Autodesk Fusion 360 part; units mm, degrees
note: some values were not read from the file. Set by a fixed rule: which sketch regions a step uses.
(part 6 of 8)
  line L4057 (-109.4829, 14.0343) -> (-108.6825, 14.0343)
  line L4058 (252.529, -8.6909) -> (249.732, -8.6909)
  line L4059 (256.681, -6.1416) -> (255.761, -6.1416)
  line L4060 (-75.345, 80.0836) -> (-76.144, 80.0836)
  line L4061 (-61.057, 41.9836) -> (-61.057, 38.8844)
  line L4062 (-108.6825, 14.0343) -> (-108.6825, 10.9337)
  line L4063 (253.129, 0.4083) -> (252.529, 0.4083)
  line L4064 (-47.283, 22.9336) -> (-48.083, 22.9336)
  line L4065 (-71.095, 67.0833) -> (-71.095, 68.0838)
  line L4066 (-65.82, 57.9344) -> (-66.62, 57.9344)
  line L4067 (-91.2764, -8.8866) -> (-91.2764, -2.6165)
  line L4068 (-148.0943, 76.9844) -> (-147.295, 76.9844)
  line L4069 (-147.295, 80.0836) -> (-148.0943, 80.0836)
  line L4070 (-56.808, 42.984) -> (-56.808, 41.9836)
  line L4071 (0.056, 81.084) -> (0.056, 80.0836)
  line L4072 (-32.482, 19.8345) -> (-32.482, 22.9336)
  line L4073 (-102.3378, -9.1167) -> (-102.3378, -8.1163)
  line L4074 (-52.045, 81.084) -> (-52.045, 80.0836)
  line L4075 (-51.532, 19.8345) -> (-51.532, 22.9336)
  line L4076 (-71.095, 68.0838) -> (-71.095, 67.0833)
  line L4077 (-147.295, 71.1844) -> (-148.0943, 71.1844)
  line L4078 (-61.057, 38.8844) -> (-61.057, 41.9836)
  line L4079 (-80.6201, 62.034) -> (-66.62, 62.034)
  line L4080 (-151.5449, 108.6602) -> (-151.5449, 105.5592)
  line L4081 (-33.283, 19.8345) -> (-32.482, 19.8345)
  line L4082 (-65.82, 52.1344) -> (-66.62, 52.1344)
  line L4083 (-151.5449, 76.9844) -> (-151.5449, 80.0836)
  line L4084 (249.732, -7.8669) -> (249.732, -8.6909)
  line L4085 (257.232, 0.4083) -> (256.23, 0.4083)
  line L4086 (-56.808, 41.9836) -> (-56.808, 42.984)
  line L4087 (-147.295, 68.0838) -> (-148.0943, 68.0838)
  line L4088 (-166.345, 99.7592) -> (-167.1443, 99.7592)
  line L4089 (-71.3829, 19.8345) -> (-71.3829, 14.0343)
  line L4090 (-66.62, 52.1344) -> (-66.62, 57.9344)
  line L4091 (-61.057, 41.9836) -> (-61.858, 41.9836)
  line L4092 (-66.62, 49.0338) -> (-66.62, 48.0333)
  line L4093 (-91.2764, 0.1836) -> (-92.1019, 0.1836)
  line L4094 (-89.551, 4.3343) -> (-89.551, 3.4138)
  line L4095 (-18.994, 71.1844) -> (-18.195, 71.1844)
  line L4096 (-123.4826, 10.9337) -> (-123.4826, 9.9333)
  line L4097 (-76.144, 68.0838) -> (-75.345, 68.0838)
  line L4098 (247.929, 0.4083) -> (247.929, -1.1159)
  line L4099 (-23.758, 42.984) -> (-37.758, 42.984)
  line L4100 (-13.945, 71.1844) -> (-13.945, 76.9844)
  line L4101 (255.761, -1.1159) -> (255.761, -2.8412)
  line L4102 (-127.7325, 14.0343) -> (-127.7325, 10.9337)
  line L4103 (249.732, -8.6909) -> (249.732, -7.8669)
  line L4104 (-147.295, 76.9844) -> (-148.0943, 76.9844)
  line L4105 (-52.333, 22.9336) -> (-52.333, 23.934)
  line L4106 (-48.083, 22.9336) -> (-48.083, 19.8345)
  line L4107 (-148.0943, 71.1844) -> (-147.295, 71.1844)
  arc A65 (-161.6635, 120.9832) -> (-163.6635, 118.9832) centre (-161.6635, 118.9832) ccw
  line L4108 (-102.3378, 4.8841) -> (-102.3378, 3.8837)
  line L4109 (-65.82, 57.9344) -> (-65.82, 61.0336)
  line L4110 (-75.345, 80.0836) -> (-75.345, 76.9844)
  line L4111 (-56.808, 33.0844) -> (-56.808, 38.8844)
  line L4112 (-171.0689, 114.1832) -> (-165.6635, 114.1832)
  line L4113 (-80.6201, 61.0336) -> (-80.6201, 62.034)
  line L4114 (-128.5329, 10.9337) -> (-127.7325, 10.9337)
  line L4115 (-66.62, 48.0333) -> (-66.62, 49.0338)
  line L4116 (-166.345, 108.6602) -> (-167.1443, 108.6602)
  line L4117 (-151.5449, 80.0836) -> (-151.5449, 76.9844)
  line L4118 (-167.1443, 105.5592) -> (-167.1443, 108.6602)
  line L4119 (-61.858, 33.0844) -> (-61.057, 33.0844)
  line L4120 (-18.195, 71.1844) -> (-18.994, 71.1844)
  line L4121 (-75.345, 68.0838) -> (-76.144, 68.0838)
  line L4122 (-152.3441, 67.0833) -> (-166.345, 67.0833)
  line L4123 (-109.4829, 9.9333) -> (-109.4829, 10.9337)
  line L4124 (-89.551, -8.8866) -> (-91.2764, -8.8866)
  line L4125 (-71.095, 71.1844) -> (-71.8941, 71.1844)
  line L4126 (-66.62, 61.0336) -> (-65.82, 61.0336)
  line L4127 (-66.62, 62.034) -> (-66.62, 61.0336)
  line L4128 (-123.4826, 9.9333) -> (-109.4829, 9.9333)
  line L4129 (-66.62, 57.9344) -> (-65.82, 57.9344)
  line L4130 (-71.095, 80.0836) -> (-71.8941, 80.0836)
  line L4131 (-167.1443, 99.7592) -> (-166.345, 99.7592)
  line L4132 (-18.195, 68.0838) -> (-18.994, 68.0838)
  line L4133 (-101.5387, 0.7845) -> (-101.5387, 3.8837)
  line L4134 (-102.3378, 0.7845) -> (-101.5387, 0.7845)
  line L4135 (252.529, 0.4083) -> (253.129, 0.4083)
  line L4136 (-18.994, 71.1844) -> (-18.994, 76.9844)
  line L4137 (-124.283, 14.0343) -> (-123.4826, 14.0343)
  line L4138 (-37.758, 28.9833) -> (-23.758, 28.9833)
  line L4139 (256.23, -0.391) -> (253.129, -0.391)
  line L4140 (-61.858, 41.9836) -> (-61.858, 42.984)
  line L4141 (-166.345, 95.6582) -> (-166.345, 96.6592)
  line L4142 (-61.858, 38.8844) -> (-61.057, 38.8844)
  line L4143 (-166.345, 109.6602) -> (-166.345, 108.6602)
  line L4144 (-23.758, 28.9833) -> (-37.758, 28.9833)
  line L4145 (-14.744, 68.0838) -> (-13.945, 68.0838)
  line L4146 (-56.808, 41.9836) -> (-57.608, 41.9836)
  line L4147 (-167.1443, 99.7592) -> (-167.1443, 96.6592)
  line L4148 (-91.2764, -2.6165) -> (-92.1019, -2.6165)
  line L4149 (-66.333, 19.8345) -> (-66.333, 14.0343)
  line L4150 (-75.345, 71.1844) -> (-75.345, 68.0838)
  line L4151 (-37.758, 42.984) -> (-23.758, 42.984)
  line L4152 (-18.994, 68.0838) -> (-18.195, 68.0838)
  line L4153 (-108.6825, 10.9337) -> (-108.6825, 14.0343)
  line L4154 (-123.4826, 14.0343) -> (-124.283, 14.0343)
  line L4155 (-66.62, 52.1344) -> (-65.82, 52.1344)
  line L4156 (-56.808, 38.8844) -> (-56.808, 33.0844)
  line L4157 (-76.144, 68.0838) -> (-76.144, 67.0833)
  line L4158 (-163.6635, 118.9832) -> (-163.6635, 116.1832)
  line L4159 (-166.345, 108.6602) -> (-166.345, 109.6602)
  line L4160 (-57.608, 33.0844) -> (-56.808, 33.0844)
  arc A66 (-165.6635, 114.1832) -> (-163.6635, 116.1832) centre (-165.6635, 116.1832) ccw
  line L4161 (-152.3441, 68.0838) -> (-151.5449, 68.0838)
  line L4162 (-52.333, 19.8345) -> (-52.333, 14.0343)
  line L4163 (-66.62, 49.0338) -> (-65.82, 49.0338)
  line L4164 (-18.195, 76.9844) -> (-18.195, 80.0836)
  line L4165 (-18.195, 80.0836) -> (-18.195, 76.9844)
  line L4166 (-127.7325, 10.9337) -> (-127.7325, 14.0343)
  line L4167 (-71.3829, 14.0343) -> (-71.3829, 19.8345)
  line L4168 (-56.808, 38.8844) -> (-57.608, 38.8844)
  line L4169 (-71.8941, 76.9844) -> (-71.8941, 80.0836)
  line L4170 (-166.345, 96.6592) -> (-166.345, 95.6582)
  line L4171 (-102.3378, 3.8837) -> (-102.3378, 4.8841)
  line L4172 (-102.3378, -5.0157) -> (-101.5387, -5.0157)
  line L4173 (-124.283, 10.9337) -> (-123.4826, 10.9337)
  line L4174 (-75.345, 71.1844) -> (-76.144, 71.1844)
  line L4175 (-123.4826, 10.9337) -> (-124.283, 10.9337)
  line L4176 (-71.8941, 68.0838) -> (-71.095, 68.0838)
  line L4177 (-66.62, 61.0336) -> (-66.62, 62.034)
  line L4178 (-102.3378, -5.0157) -> (-102.3378, 0.7845)
  line L4179 (-9.469, 105.5592) -> (-8.67, 105.5592)
  line L4180 (-90.4329, 14.0343) -> (-90.4329, 19.8345)
  line L4181 (-9.469, 52.1344) -> (-9.469, 57.9344)
  line L4182 (5.105, 68.0838) -> (4.306, 68.0838)
  line L4183 (-42.007, 38.8844) -> (-42.808, 38.8844)
  line L4184 (243.459, -2.8412) -> (242.482, -2.8412)
  line L4185 (-9.469, 108.6602) -> (-9.469, 109.6602)
  line L4186 (-104.4326, 9.9333) -> (-90.4329, 9.9333)
  line L4187 (-146.7824, 49.0338) -> (-146.7824, 52.1344)
  line L4188 (256.23, 14.4091) -> (257.232, 14.4091)
  line L4189 (-128.2451, 108.6602) -> (-129.0441, 108.6602)
  line L4190 (-90.4329, 14.0343) -> (-89.6325, 14.0343)
  line L4191 (-8.67, 105.5592) -> (-9.469, 105.5592)
  line L4192 (-128.2451, 96.6592) -> (-128.2451, 95.6582)
  line L4193 (-147.583, 57.9344) -> (-146.7824, 57.9344)
  line L4194 (253.129, 15.2084) -> (256.23, 15.2084)
  line L4195 (256.23, 15.2084) -> (253.129, 15.2084)
  line L4196 (-52.333, 9.9333) -> (-66.333, 9.9333)
  line L4197 (244.232, 0.4083) -> (244.232, -0.391)
  line L4198 (-128.2451, 95.6582) -> (-128.2451, 96.6592)
  line L4199 (0.855, 71.1844) -> (0.855, 68.0838)
  line L4200 (0.056, 81.084) -> (-13.945, 81.084)
  line L4201 (242.482, -6.1416) -> (242.482, -2.8412)
  line L4202 (-147.583, 52.1344) -> (-147.583, 57.9344)
  line L4203 (-71.095, 67.0833) -> (-57.094, 67.0833)
  line L4204 (-9.469, 52.1344) -> (-8.67, 52.1344)
  line L4205 (-146.7824, 52.1344) -> (-146.7824, 49.0338)
  line L4206 (252.529, 15.9333) -> (255.761, 15.9333)
  line L4207 (-42.808, 42.984) -> (-42.808, 41.9836)
  line L4208 (-42.808, 28.9833) -> (-42.808, 29.9838)
  line L4209 (244.232, -0.391) -> (247.333, -0.391)
  line L4210 (-128.2451, 99.7592) -> (-129.0441, 99.7592)
  line L4211 (-44.901, -4.4162) -> (-84.5267, -4.4162)
  line L4212 (-90.4329, 10.9337) -> (-90.4329, 9.9333)
  line L4213 (5.105, 71.1844) -> (4.306, 71.1844)
  line L4214 (-9.469, 61.0336) -> (-8.67, 61.0336)
  line L4215 (-116.3388, 4.8841) -> (-102.3378, 4.8841)
  line L4216 (-42.007, 29.9838) -> (-42.808, 29.9838)
  line L4217 (-128.2451, 96.6592) -> (-129.0441, 96.6592)
  line L4218 (238.979, -5.0157) -> (238.182, -5.0157)
  line L4219 (5.105, 68.0838) -> (5.105, 67.0833)
  line L4220 (-90.4329, 9.9333) -> (-104.4326, 9.9333)
  line L4221 (-57.094, 81.084) -> (-71.095, 81.084)
  line L4222 (-8.67, 61.0336) -> (-9.469, 61.0336)
  line L4223 (243.459, -1.1159) -> (247.929, -1.1159)
  line L4224 (255.761, 15.9333) -> (252.529, 15.9333)
  line L4225 (-42.808, 33.0844) -> (-42.007, 33.0844)
  line L4226 (-90.4329, 10.9337) -> (-89.6325, 10.9337)
  line L4227 (-147.583, 52.1344) -> (-146.7824, 52.1344)
  line L4228 (-105.233, 10.9337) -> (-105.233, 14.0343)
  line L4229 (-129.0441, 108.6602) -> (-128.2451, 108.6602)
  line L4230 (-129.0441, 99.7592) -> (-128.2451, 99.7592)
  line L4231 (-133.294, 67.0833) -> (-147.295, 67.0833)
  line L4232 (-147.583, 62.034) -> (-147.583, 61.0336)
  line L4233 (-146.7824, 61.0336) -> (-147.583, 61.0336)
  line L4234 (5.105, 80.0836) -> (4.306, 80.0836)
  line L4235 (-57.094, 67.0833) -> (-71.095, 67.0833)
  line L4236 (-8.67, 57.9344) -> (-9.469, 57.9344)
  line L4237 (243.459, -6.1416) -> (242.482, -6.1416)
  line L4238 (-42.808, 29.9838) -> (-42.808, 28.9833)
  line L4239 (252.529, 14.4091) -> (253.129, 14.4091)
  line L4240 (5.105, 80.0836) -> (5.105, 81.084)
  line L4241 (-116.3388, -9.1167) -> (-102.3378, -9.1167)
  line L4242 (-42.007, 41.9836) -> (-42.808, 41.9836)
  line L4243 (-146.7824, 57.9344) -> (-146.7824, 61.0336)
  line L4244 (242.482, -2.8412) -> (243.459, -2.8412)
  line L4245 (-129.0441, 96.6592) -> (-128.2451, 96.6592)
  line L4246 (244.232, -0.391) -> (244.232, 0.4083)
  line L4247 (-102.3378, -9.1167) -> (-116.3388, -9.1167)
  line L4248 (243.459, -1.1159) -> (243.459, -2.8412)
  line L4249 (-104.4326, 10.9337) -> (-105.233, 10.9337)
  line L4250 (238.182, -5.0157) -> (238.182, 0.7845)
  line L4251 (-146.7824, 52.1344) -> (-147.583, 52.1344)
  line L4252 (-42.808, 38.8844) -> (-42.808, 33.0844)
  line L4253 (238.979, -8.1163) -> (238.182, -8.1163)
  line L4254 (-129.0441, 99.7592) -> (-129.0441, 96.6592)
  line L4255 (-128.2451, 105.5592) -> (-129.0441, 105.5592)
  line L4256 (-89.6325, 10.9337) -> (-89.6325, 14.0343)
  line L4257 (-90.4329, 9.9333) -> (-90.4329, 10.9337)
  line L4258 (242.482, -2.8412) -> (242.482, -6.1416)
  line L4259 (-128.2451, 99.7592) -> (-128.2451, 105.5592)
  line L4260 (-128.2451, 108.6602) -> (-128.2451, 109.6602)
  line L4261 (-146.7824, 61.0336) -> (-146.7824, 57.9344)
  line L4262 (5.105, 81.084) -> (5.105, 80.0836)
  line L4263 (-42.007, 33.0844) -> (-42.808, 33.0844)
  line L4264 (238.182, -8.1163) -> (238.182, -9.1167)
  line L4265 (-42.808, 33.0844) -> (-42.808, 38.8844)
  line L4266 (0.855, 76.9844) -> (0.855, 80.0836)
  line L4267 (-147.295, 67.0833) -> (-133.294, 67.0833)
  line L4268 (-71.095, 81.084) -> (-57.094, 81.084)
  line L4269 (-147.583, 48.0333) -> (-147.583, 49.0338)
  line L4270 (-9.469, 57.9344) -> (-8.67, 57.9344)
  line L4271 (-57.094, 68.0838) -> (-57.094, 67.0833)
  line L4272 (-52.844, 76.9844) -> (-52.045, 76.9844)
  line L4273 (-147.583, 61.0336) -> (-146.7824, 61.0336)
  line L4274 (-166.345, 109.6602) -> (-152.3441, 109.6602)
  line L4275 (-129.0441, 96.6592) -> (-129.0441, 99.7592)
  line L4276 (-104.4326, 14.0343) -> (-105.233, 14.0343)
  line L4277 (-147.295, 81.084) -> (-133.294, 81.084)
  line L4278 (-129.0441, 105.5592) -> (-129.0441, 108.6602)
  line L4279 (0.056, 76.9844) -> (0.855, 76.9844)
  line L4280 (-52.844, 80.0836) -> (-52.045, 80.0836)
  line L4281 (253.129, -0.391) -> (253.129, 0.4083)
  line L4282 (-128.2451, 105.5592) -> (-128.2451, 99.7592)
  line L4283 (-84.5267, -4.4162) -> (-44.901, -4.4162)
  line L4284 (-162.3832, 57.9344) -> (-162.3832, 61.0336)
  line L4285 (-57.094, 76.9844) -> (-57.094, 71.1844)
  line L4286 (-57.094, 67.0833) -> (-57.094, 68.0838)
  line L4287 (-133.294, 81.084) -> (-147.295, 81.084)
  line L4288 (-162.3832, 52.1344) -> (-162.3832, 49.0338)
  line L4289 (-162.3832, 61.0336) -> (-162.3832, 57.9344)
  line L4290 (-128.2451, 109.6602) -> (-128.2451, 108.6602)
  line L4291 (-129.0441, 108.6602) -> (-129.0441, 105.5592)
  line L4292 (244.232, 0.4083) -> (243.23, 0.4083)
  line L4293 (-89.6325, 14.0343) -> (-89.6325, 10.9337)
  line L4294 (-52.844, 76.9844) -> (-52.844, 80.0836)
  line L4295 (247.333, -0.391) -> (244.232, -0.391)
  line L4296 (-89.6325, 14.0343) -> (-90.4329, 14.0343)
  line L4297 (-152.3441, 109.6602) -> (-152.3441, 108.6602)
  line L4298 (-162.3832, 49.0338) -> (-162.3832, 52.1344)
  line L4299 (-8.67, 57.9344) -> (-8.67, 61.0336)
  line L4300 (-105.233, 14.0343) -> (-104.4326, 14.0343)
  line L4301 (-151.5449, 96.6592) -> (-151.5449, 99.7592)
  line L4302 (238.182, 4.8841) -> (238.182, 3.8837)
  line L4303 (238.182, 0.7845) -> (238.182, -5.0157)
  line L4304 (-152.3441, 105.5592) -> (-151.5449, 105.5592)
  line L4305 (-152.3441, 96.6592) -> (-152.3441, 95.6582)
  line L4306 (-52.844, 71.1844) -> (-52.844, 68.0838)
  line L4307 (242.482, -6.1416) -> (243.459, -6.1416)
  line L4308 (4.306, 71.1844) -> (5.105, 71.1844)
  line L4309 (-162.3832, 52.1344) -> (-161.5825, 52.1344)
  line L4310 (0.056, 67.0833) -> (0.056, 68.0838)
  line L4311 (243.459, -6.1416) -> (243.459, -7.8669)
  line L4312 (0.056, 71.1844) -> (0.855, 71.1844)
  line L4313 (-9.469, 62.034) -> (-9.469, 61.0336)
  line L4314 (243.459, -2.8412) -> (243.459, -1.1159)
  line L4315 (-152.3441, 80.0836) -> (-152.3441, 81.084)
  line L4316 (238.979, 0.7845) -> (238.182, 0.7845)
  line L4317 (4.306, 68.0838) -> (5.105, 68.0838)
  line L4318 (-161.5825, 61.0336) -> (-162.3832, 61.0336)
  line L4319 (238.182, 3.8837) -> (238.979, 3.8837)
  line L4320 (-152.3441, 105.5592) -> (-152.3441, 99.7592)
  line L4321 (-57.094, 76.9844) -> (-56.295, 76.9844)
  line L4322 (-162.3832, 49.0338) -> (-161.5825, 49.0338)
  line L4323 (-52.844, 71.1844) -> (-52.045, 71.1844)
  line L4324 (-52.045, 80.0836) -> (-52.844, 80.0836)
  line L4325 (-151.5449, 108.6602) -> (-152.3441, 108.6602)
  line L4326 (255.761, -6.1416) -> (256.681, -6.1416)
  line L4327 (-151.5449, 105.5592) -> (-151.5449, 108.6602)
  line L4328 (256.681, -2.8412) -> (255.761, -2.8412)
  line L4329 (-9.469, 61.0336) -> (-9.469, 62.034)
  line L4330 (-161.5825, 49.0338) -> (-162.3832, 49.0338)
  line L4331 (-162.3832, 57.9344) -> (-161.5825, 57.9344)
  line L4332 (-57.094, 81.084) -> (-57.094, 80.0836)
  line L4333 (243.23, 0.4083) -> (244.232, 0.4083)
  line L4334 (-9.469, 57.9344) -> (-9.469, 52.1344)
  line L4335 (-56.295, 68.0838) -> (-56.295, 71.1844)
  line L4336 (-161.5825, 61.0336) -> (-161.5825, 62.034)
  line L4337 (238.979, -5.0157) -> (238.979, -8.1163)
  line L4338 (238.979, -8.1163) -> (238.979, -5.0157)
  line L4339 (-152.3441, 95.6582) -> (-152.3441, 96.6592)
  line L4340 (252.529, -8.6909) -> (252.529, -7.8669)
  line L4341 (4.306, 80.0836) -> (4.306, 76.9844)
  line L4342 (-152.3441, 96.6592) -> (-151.5449, 96.6592)
  line L4343 (-161.5825, 52.1344) -> (-162.3832, 52.1344)
  line L4344 (243.459, -7.8669) -> (243.459, -6.1416)
  line L4345 (-151.5449, 96.6592) -> (-152.3441, 96.6592)
  line L4346 (-161.5825, 57.9344) -> (-161.5825, 52.1344)
  line L4347 (-56.295, 71.1844) -> (-57.094, 71.1844)
  line L4348 (255.761, -7.8669) -> (255.761, -6.1416)
  line L4349 (238.979, 3.8837) -> (238.182, 3.8837)
  line L4350 (-151.5449, 71.1844) -> (-152.3441, 71.1844)
  line L4351 (-161.5825, 62.034) -> (-147.583, 62.034)
  line L4352 (-52.045, 76.9844) -> (-52.045, 71.1844)
  line L4353 (-52.333, 23.934) -> (-52.333, 22.9336)
  line L4354 (-147.583, 48.0333) -> (-161.5825, 48.0333)
  line L4355 (-166.345, 95.6582) -> (-152.3441, 95.6582)
  line L4356 (-52.045, 71.1844) -> (-52.844, 71.1844)
  line L4357 (238.182, -5.0157) -> (238.979, -5.0157)
  line L4358 (4.306, 76.9844) -> (5.105, 76.9844)
  line L4359 (-161.5825, 48.0333) -> (-147.583, 48.0333)
  line L4360 (238.979, 3.8837) -> (238.979, 0.7845)
  line L4361 (-152.3441, 95.6582) -> (-166.345, 95.6582)
  line L4362 (252.529, -7.8669) -> (255.761, -7.8669)
  line L4363 (-145.2635, 118.9832) -> (-145.2635, 116.1832)
  line L4364 (247.929, 0.4083) -> (247.333, 0.4083)
  line L4365 (256.23, 0.4083) -> (256.23, -0.391)
  line L4366 (-51.532, 19.8345) -> (-52.333, 19.8345)
  line L4367 (0.855, 68.0838) -> (0.855, 71.1844)
  line L4368 (-147.583, 62.034) -> (-161.5825, 62.034)
  line L4369 (-151.5449, 105.5592) -> (-152.3441, 105.5592)
  line L4370 (-47.283, 23.934) -> (-47.283, 22.9336)
  line L4371 (247.333, 0.4083) -> (247.929, 0.4083)
  line L4372 (-161.5825, 49.0338) -> (-161.5825, 48.0333)
  line L4373 (4.306, 80.0836) -> (5.105, 80.0836)
  line L4374 (-57.094, 80.0836) -> (-57.094, 81.084)
  line L4375 (-51.532, 22.9336) -> (-51.532, 19.8345)
  line L4376 (-161.5825, 57.9344) -> (-162.3832, 57.9344)
  line L4377 (4.306, 68.0838) -> (4.306, 71.1844)
  line L4378 (-152.3441, 80.0836) -> (-151.5449, 80.0836)
  line L4379 (-32.482, 22.9336) -> (-32.482, 19.8345)
  line L4380 (-52.844, 80.0836) -> (-52.844, 76.9844)
  line L4381 (-66.333, 9.9333) -> (-52.333, 9.9333)
  line L4382 (-161.5825, 48.0333) -> (-161.5825, 49.0338)
  line L4383 (-156.5635, 120.9832) -> (-157.3635, 120.9832)
  line L4384 (0.056, 71.1844) -> (0.056, 76.9844)
  line L4385 (-52.045, 68.0838) -> (-52.844, 68.0838)
  arc A67 (-145.2635, 116.1832) -> (-143.2635, 114.1832) centre (-143.2635, 116.1832) ccw
  line L4386 (-162.3832, 61.0336) -> (-161.5825, 61.0336)
  line L4387 (-148.0943, 68.0838) -> (-147.295, 68.0838)
  line L4388 (-147.2635, 120.9832) -> (-161.6635, 120.9832)
  line L4389 (5.105, 67.0833) -> (5.105, 68.0838)
  line L4390 (252.529, -1.1159) -> (252.529, 0.4083)
  line L4391 (256.681, -6.1416) -> (256.681, -2.8412)
  line L4392 (253.129, -0.391) -> (256.23, -0.391)
  line L4393 (-56.295, 68.0838) -> (-57.094, 68.0838)
  line L4394 (5.105, 76.9844) -> (5.105, 71.1844)
  line L4395 (255.761, -2.8412) -> (255.761, -1.1159)
  line L4396 (-47.283, 19.8345) -> (-48.083, 19.8345)
  line L4397 (-80.6201, 57.9344) -> (-81.4205, 57.9344)
  line L4398 (0.855, 68.0838) -> (0.056, 68.0838)
  line L4399 (256.23, 0.4083) -> (257.232, 0.4083)
  line L4400 (-161.5825, 52.1344) -> (-161.5825, 57.9344)
  line L4401 (-52.844, 68.0838) -> (-52.045, 68.0838)
  line L4402 (-33.283, 22.9336) -> (-32.482, 22.9336)
  line L4403 (-101.5387, 3.8837) -> (-101.5387, 0.7845)
  line L4404 (-152.3441, 109.6602) -> (-166.345, 109.6602)
  line L4405 (-152.3441, 108.6602) -> (-152.3441, 109.6602)
  line L4406 (0.855, 80.0836) -> (0.855, 76.9844)
  line L4407 (-147.295, 67.0833) -> (-147.295, 68.0838)
  line L4408 (-52.333, 19.8345) -> (-51.532, 19.8345)
  line L4409 (-52.045, 80.0836) -> (-52.045, 81.084)
  line L4410 (-52.045, 76.9844) -> (-52.844, 76.9844)
  line L4411 (-89.551, -9.8664) -> (-89.551, -8.8866)
  line L4412 (-52.333, 22.9336) -> (-51.532, 22.9336)
  line L4413 (-56.295, 80.0836) -> (-57.094, 80.0836)
  line L4414 (252.529, 0.4083) -> (252.529, -1.1159)
  line L4415 (256.681, -2.8412) -> (256.681, -6.1416)
  line L4416 (5.105, 76.9844) -> (4.306, 76.9844)
  line L4417 (5.105, 71.1844) -> (5.105, 76.9844)
  line L4418 (-147.295, 81.084) -> (-147.295, 80.0836)
  line L4419 (-56.295, 76.9844) -> (-56.295, 80.0836)
  line L4420 (247.333, 0.4083) -> (247.333, -0.391)
  line L4421 (-92.1019, -2.6165) -> (-91.2764, -2.6165)
  line L4422 (-89.551, -8.8866) -> (-89.551, -9.8664)
  line L4423 (-151.5449, 99.7592) -> (-152.3441, 99.7592)
  line L4424 (-161.5825, 62.034) -> (-161.5825, 61.0336)
  line L4425 (-151.5449, 71.1844) -> (-151.5449, 68.0838)
  circle A68 centre (-156.9635, 117.5832) radius 1.7
  line L4426 (-13.945, 67.0833) -> (0.056, 67.0833)
  line L4427 (252.529, -1.1159) -> (255.761, -1.1159)
  line L4428 (-102.3378, 4.8841) -> (-116.3388, 4.8841)
  line L4429 (-33.283, 22.9336) -> (-33.283, 23.934)
  line L4430 (0.056, 76.9844) -> (0.056, 71.1844)
  line L4431 (-48.083, 22.9336) -> (-47.283, 22.9336)
  line L4432 (-147.295, 76.9844) -> (-147.295, 71.1844)
  circle A69 centre (-156.9635, 117.5832) radius 1.7
  line L4433 (-47.283, 14.0343) -> (-48.083, 14.0343)
  line L4434 (-32.482, 14.0343) -> (-32.482, 10.9337)
  line L4435 (-52.333, 9.9333) -> (-52.333, 10.9337)
  line L4436 (-45.702, -8.1163) -> (-44.901, -8.1163)
  line L4437 (-44.901, 3.8837) -> (-44.901, 4.8841)
  line L4438 (-44.901, -8.1163) -> (-44.901, -9.1167)
  line L4439 (-48.083, 14.0343) -> (-47.283, 14.0343)
  line L4440 (-45.702, 0.7845) -> (-44.901, 0.7845)
  line L4441 (-32.482, 10.9337) -> (-33.283, 10.9337)
  line L4442 (-45.702, -8.1163) -> (-45.702, -5.0157)
  line L4443 (-32.482, 14.0343) -> (-33.283, 14.0343)
  line L4444 (-48.083, 14.0343) -> (-48.083, 10.9337)
  line L4445 (-44.901, 3.8837) -> (-45.702, 3.8837)
  line L4446 (-44.901, -4.4162) -> (-44.901, -5.0157)
  line L4447 (-45.702, -5.0157) -> (-45.702, -8.1163)
  line L4448 (-44.901, 4.8841) -> (-44.901, 3.8837)
  line L4449 (-48.083, 10.9337) -> (-48.083, 14.0343)
  line L4450 (-44.901, 0.1836) -> (-44.901, 0.7845)
  line L4451 (-44.901, 0.7845) -> (-44.901, 0.1836)
  line L4452 (-45.702, 0.7845) -> (-45.702, 3.8837)
  line L4453 (-61.858, 38.8844) -> (-61.858, 33.0844)
  line L4454 (-61.858, 42.984) -> (-61.858, 41.9836)
  line L4455 (-102.3378, -8.1163) -> (-101.5387, -8.1163)
  line L4456 (-101.5387, 0.7845) -> (-102.3378, 0.7845)
  line L4457 (-166.345, 99.7592) -> (-166.345, 105.5592)
  line L4458 (-13.945, 68.0838) -> (-14.744, 68.0838)
  line L4459 (-61.858, 41.9836) -> (-61.057, 41.9836)
  line L4460 (-166.345, 76.9844) -> (-166.345, 71.1844)
  line L4461 (-76.144, 71.1844) -> (-75.345, 71.1844)
  line L4462 (-61.057, 33.0844) -> (-61.858, 33.0844)
  line L4463 (-166.345, 80.0836) -> (-166.345, 81.084)
  line L4464 (-123.4826, 9.9333) -> (-123.4826, 10.9337)
  line L4465 (-166.345, 81.084) -> (-166.345, 80.0836)
  line L4466 (-109.4829, 9.9333) -> (-123.4826, 9.9333)
  line L4467 (-13.945, 76.9844) -> (-13.945, 71.1844)
  line L4468 (-76.144, 80.0836) -> (-76.144, 81.084)
  line L4469 (-14.744, 68.0838) -> (-14.744, 71.1844)
  line L4470 (-66.333, 14.0343) -> (-66.333, 19.8345)
  line L4471 (-126.1517, -5.0157) -> (-126.1517, 0.7845)
  line L4472 (-166.345, 105.5592) -> (-166.345, 99.7592)
  line L4473 (-167.1443, 96.6592) -> (-166.345, 96.6592)
  line L4474 (-125.3512, 3.8837) -> (-125.3512, 0.7845)
  line L4475 (-125.3512, 3.8837) -> (-126.1517, 3.8837)
  line L4476 (-166.345, 67.0833) -> (-152.3441, 67.0833)
  line L4477 (-57.608, 41.9836) -> (-57.608, 38.8844)
  line L4478 (-91.2764, 3.4138) -> (-91.2764, 0.1836)
  line L4479 (-13.945, 68.0838) -> (-13.945, 67.0833)
  line L4480 (-92.1019, 0.1836) -> (-92.1019, -2.6165)
  line L4481 (-80.6201, 62.034) -> (-80.6201, 61.0336)
  line L4482 (-167.1443, 105.5592) -> (-166.345, 105.5592)
  line L4483 (-151.5449, 76.9844) -> (-152.3441, 76.9844)
  line L4484 (-127.7325, 14.0343) -> (-128.5329, 14.0343)
  line L4485 (-101.5387, 3.8837) -> (-102.3378, 3.8837)
  line L4486 (-76.144, 71.1844) -> (-76.144, 76.9844)
  line L4487 (-13.945, 81.084) -> (0.056, 81.084)
  line L4488 (-80.6201, 48.0333) -> (-66.62, 48.0333)
  line L4489 (-13.945, 80.0836) -> (-14.744, 80.0836)
  line L4490 (-128.5329, 10.9337) -> (-128.5329, 9.9333)
  line L4491 (-124.283, 14.0343) -> (-124.283, 10.9337)
  line L4492 (-75.345, 76.9844) -> (-76.144, 76.9844)
  line L4493 (-61.057, 38.8844) -> (-61.858, 38.8844)
  line L4494 (-166.345, 96.6592) -> (-167.1443, 96.6592)
  line L4495 (-166.345, 76.9844) -> (-167.1443, 76.9844)
  line L4496 (-167.1443, 108.6602) -> (-167.1443, 105.5592)
  line L4497 (-109.4829, 10.9337) -> (-108.6825, 10.9337)
  line L4498 (-128.5329, 14.0343) -> (-127.7325, 14.0343)
  line L4499 (-167.1443, 108.6602) -> (-166.345, 108.6602)
  line L4500 (-101.5387, -5.0157) -> (-102.3378, -5.0157)
  line L4501 (-56.808, 33.0844) -> (-57.608, 33.0844)
  line L4502 (-126.1517, -5.0157) -> (-125.3512, -5.0157)
  line L4503 (-109.4829, 10.9337) -> (-109.4829, 9.9333)
  line L4504 (-76.144, 80.0836) -> (-75.345, 80.0836)
  line L4505 (-76.144, 81.084) -> (-76.144, 80.0836)
  line L4506 (-91.2764, -8.8866) -> (-89.551, -8.8866)
  line L4507 (-117.1378, -8.1163) -> (-116.3388, -8.1163)
  line L4508 (-117.1378, 0.7845) -> (-116.3388, 0.7845)
  line L4509 (-167.1443, 96.6592) -> (-167.1443, 99.7592)
  line L4510 (-57.608, 38.8844) -> (-56.808, 38.8844)
  line L4511 (-71.095, 76.9844) -> (-71.8941, 76.9844)
  line L4512 (-18.994, 76.9844) -> (-18.195, 76.9844)
  line L4513 (-102.3378, -8.1163) -> (-102.3378, -9.1167)
  line L4514 (-13.945, 81.084) -> (-13.945, 80.0836)
  line L4515 (-89.551, 3.4138) -> (-89.551, 4.3343)
  line L4516 (-167.1443, 80.0836) -> (-167.1443, 76.9844)
  line L4517 (-14.744, 80.0836) -> (-13.945, 80.0836)
  line L4518 (-167.1443, 76.9844) -> (-167.1443, 80.0836)
  line L4519 (-57.608, 38.8844) -> (-57.608, 41.9836)
  line L4520 (-128.5329, 9.9333) -> (-128.5329, 10.9337)
  line L4521 (-47.283, 19.8345) -> (-47.283, 14.0343)
  line L4522 (0.056, 80.0836) -> (0.855, 80.0836)
  line L4523 (-18.994, 80.0836) -> (-18.195, 80.0836)
  line L4524 (-125.3512, -8.1163) -> (-126.1517, -8.1163)
  line L4525 (-125.3512, 0.7845) -> (-126.1517, 0.7845)
  line L4526 (-57.608, 41.9836) -> (-56.808, 41.9836)
  line L4527 (-85.3826, 14.0343) -> (-85.3826, 19.8345)
  line L4528 (-101.5387, -8.1163) -> (-101.5387, -5.0157)
  line L4529 (-127.7325, 10.9337) -> (-128.5329, 10.9337)
  line L4530 (-85.6704, 49.0338) -> (-84.87, 49.0338)
  line L4531 (-71.095, 80.0836) -> (-71.095, 81.084)
  line L4532 (-71.8941, 71.1844) -> (-71.095, 71.1844)
  line L4533 (-71.8941, 68.0838) -> (-71.8941, 71.1844)
  line L4534 (-75.345, 76.9844) -> (-75.345, 80.0836)
  line L4535 (-61.858, 33.0844) -> (-61.858, 38.8844)
  line L4536 (-33.283, 14.0343) -> (-33.283, 19.8345)
  line L4537 (-71.8941, 76.9844) -> (-71.095, 76.9844)
  line L4538 (-166.345, 105.5592) -> (-167.1443, 105.5592)
  line L4539 (-18.195, 71.1844) -> (-18.195, 68.0838)
  line L4540 (-166.345, 81.084) -> (-152.3441, 81.084)
  line L4541 (-166.345, 68.0838) -> (-167.1443, 68.0838)
  line L4542 (-167.1443, 76.9844) -> (-166.345, 76.9844)
  line L4543 (-163.3635, 114.1832) -> (-165.0689, 114.1832)
  line L4544 (-85.6704, 48.0333) -> (-85.6704, 49.0338)
  line L4545 (-124.283, 10.9337) -> (-124.283, 14.0343)
  line L4546 (-18.994, 67.0833) -> (-18.994, 68.0838)
  line L4547 (-28.233, 14.0343) -> (-28.233, 19.8345)
  line L4548 (-84.87, 61.0336) -> (-85.6704, 61.0336)
  line L4549 (-71.095, 68.0838) -> (-71.8941, 68.0838)
  line L4550 (-71.095, 71.1844) -> (-71.095, 76.9844)
  line L4551 (-76.144, 67.0833) -> (-76.144, 68.0838)
  line L4552 (-29.033, 14.0343) -> (-28.233, 14.0343)
  line L4553 (-167.1443, 71.1844) -> (-167.1443, 68.0838)
  line L4554 (-84.87, 52.1344) -> (-85.6704, 52.1344)
  line L4555 (-117.1378, -5.0157) -> (-117.1378, -8.1163)
  line L4556 (-166.345, 67.0833) -> (-166.345, 68.0838)
  line L4557 (-126.1517, 3.8837) -> (-126.1517, 4.8841)
  line L4558 (-47.283, 14.0343) -> (-47.283, 19.8345)
  line L4559 (-80.6201, 57.9344) -> (-80.6201, 52.1344)
  line L4560 (-116.3388, 3.8837) -> (-116.3388, 4.8841)
  line L4561 (-18.994, 76.9844) -> (-18.994, 71.1844)
  line L4562 (0.855, 76.9844) -> (0.056, 76.9844)
  line L4563 (-80.6201, 49.0338) -> (-80.6201, 48.0333)
  line L4564 (-166.345, 68.0838) -> (-166.345, 67.0833)
  line L4565 (-13.945, 71.1844) -> (-14.744, 71.1844)
  line L4566 (-81.4205, 61.0336) -> (-80.6201, 61.0336)
  line L4567 (-116.3388, -5.0157) -> (-117.1378, -5.0157)
  line L4568 (-71.8941, 80.0836) -> (-71.095, 80.0836)
  line L4569 (-152.3441, 76.9844) -> (-151.5449, 76.9844)
  line L4570 (-29.033, 14.0343) -> (-29.033, 10.9337)
  line L4571 (-166.345, 80.0836) -> (-167.1443, 80.0836)
  line L4572 (-126.1517, 3.8837) -> (-125.3512, 3.8837)
  line L4573 (-85.3826, 19.8345) -> (-85.3826, 14.0343)
  line L4574 (-80.6201, 52.1344) -> (-80.6201, 57.9344)
  line L4575 (-14.744, 71.1844) -> (-14.744, 68.0838)
  line L4576 (-28.233, 19.8345) -> (-28.233, 14.0343)
  line L4577 (-85.6704, 61.0336) -> (-84.87, 61.0336)
  line L4578 (-28.233, 9.9333) -> (-28.233, 10.9337)
  line L4579 (-84.87, 49.0338) -> (-85.6704, 49.0338)
  line L4580 (0.056, 67.0833) -> (-13.945, 67.0833)
  line L4581 (-81.4205, 52.1344) -> (-80.6201, 52.1344)
  line L4582 (-167.1443, 68.0838) -> (-167.1443, 71.1844)
  line L4583 (0.056, 68.0838) -> (0.056, 67.0833)
  line L4584 (-126.1517, 0.7845) -> (-126.1517, -5.0157)
  line L4585 (-66.62, 62.034) -> (-80.6201, 62.034)
  line L4586 (-30.902, -8.1163) -> (-30.101, -8.1163)
  line L4587 (-84.87, 49.0338) -> (-84.87, 52.1344)
  line L4588 (-30.101, -8.1163) -> (-30.101, -5.0157)
  line L4589 (-167.1443, 80.0836) -> (-166.345, 80.0836)
  line L4590 (-28.233, 14.0343) -> (-29.033, 14.0343)
  line L4591 (-84.87, 57.9344) -> (-84.87, 61.0336)
  line L4592 (-30.902, 3.8837) -> (-30.902, 4.8841)
  line L4593 (-166.345, 71.1844) -> (-167.1443, 71.1844)
  line L4594 (-86.2521, 3.4138) -> (-86.2521, 4.3343)
  line L4595 (-75.345, 68.0838) -> (-75.345, 71.1844)
  line L4596 (-33.283, 19.8345) -> (-33.283, 14.0343)
  line L4597 (-61.858, 28.9833) -> (-75.8576, 28.9833)
  line L4598 (-117.1378, 3.8837) -> (-117.1378, 0.7845)
  line L4599 (-29.033, 10.9337) -> (-28.233, 10.9337)
  line L4600 (-125.3512, -5.0157) -> (-126.1517, -5.0157)
  line L4601 (-52.333, 14.0343) -> (-52.333, 19.8345)
  line L4602 (-30.902, -5.0157) -> (-30.101, -5.0157)
  line L4603 (-152.3441, 68.0838) -> (-152.3441, 67.0833)
  line L4604 (-18.195, 68.0838) -> (-18.195, 71.1844)
  line L4605 (-126.1517, -9.1167) -> (-126.1517, -8.1163)
  line L4606 (-126.1517, -8.1163) -> (-125.3512, -8.1163)
  line L4607 (-167.1443, 71.1844) -> (-166.345, 71.1844)
  line L4608 (-76.144, 76.9844) -> (-76.144, 71.1844)
  line L4609 (-13.945, 76.9844) -> (-14.744, 76.9844)
  line L4610 (-18.994, 80.0836) -> (-18.994, 81.084)
  line L4611 (-85.6704, 52.1344) -> (-85.6704, 57.9344)
  line L4612 (0.855, 71.1844) -> (0.056, 71.1844)
  line L4613 (-117.1378, 3.8837) -> (-116.3388, 3.8837)
  line L4614 (-84.87, 52.1344) -> (-84.87, 49.0338)
  line L4615 (-28.233, 10.9337) -> (-29.033, 10.9337)
  line L4616 (-57.608, 29.9838) -> (-56.808, 29.9838)
  line L4617 (-30.902, 0.1836) -> (-30.902, 0.7845)
  line L4618 (-14.744, 76.9844) -> (-13.945, 76.9844)
  line L4619 (-84.5267, 3.4138) -> (-86.2521, 3.4138)
  line L4620 (-116.3388, -5.0157) -> (-116.3388, 0.7845)
  line L4621 (-167.1443, 68.0838) -> (-166.345, 68.0838)
  line L4622 (-18.195, 76.9844) -> (-18.994, 76.9844)
  line L4623 (-67.133, 22.9336) -> (-67.133, 19.8345)
  line L4624 (-166.345, 71.1844) -> (-166.345, 76.9844)
  line L4625 (-61.858, 42.984) -> (-75.8576, 42.984)
  line L4626 (-126.1517, 4.8841) -> (-126.1517, 3.8837)
  line L4627 (-18.994, 68.0838) -> (-18.994, 67.0833)
  line L4628 (-67.133, 19.8345) -> (-67.133, 22.9336)
  line L4629 (-70.582, 10.9337) -> (-71.3829, 10.9337)
  line L4630 (-85.6704, 57.9344) -> (-85.6704, 52.1344)
  line L4631 (-83.201, -18.7426) -> (-83.201, -15.9426)
  line L4632 (-13.945, 67.0833) -> (-13.945, 68.0838)
  line L4633 (-66.62, 48.0333) -> (-80.6201, 48.0333)
  line L4634 (0.056, 68.0838) -> (0.855, 68.0838)
  line L4635 (-30.101, 0.7845) -> (-30.101, 3.8837)
  line L4636 (-14.744, 80.0836) -> (-14.744, 76.9844)
  line L4637 (-28.233, 10.9337) -> (-28.233, 9.9333)
  line L4638 (-125.3512, -8.1163) -> (-125.3512, -5.0157)
  line L4639 (-125.3512, -5.0157) -> (-125.3512, -8.1163)
  line L4640 (-85.6704, 61.0336) -> (-85.6704, 62.034)
  line L4641 (-75.8576, 42.984) -> (-61.858, 42.984)
  line L4642 (-66.333, 19.8345) -> (-67.133, 19.8345)
  line L4643 (-151.5449, 80.0836) -> (-152.3441, 80.0836)
  line L4644 (-85.6704, 62.034) -> (-85.6704, 61.0336)
  line L4645 (-85.6704, 49.0338) -> (-85.6704, 48.0333)
  line L4646 (-30.101, -5.0157) -> (-30.101, -8.1163)
  line L4647 (-126.1517, -8.1163) -> (-126.1517, -9.1167)
  arc A70 (-85.201, -20.7426) -> (-83.201, -18.7426) centre (-85.201, -18.7426) ccw
  line L4648 (-67.133, 10.9337) -> (-67.133, 14.0343)
  line L4649 (-152.3441, 81.084) -> (-152.3441, 80.0836)
  line L4650 (-61.057, 33.0844) -> (-61.057, 29.9838)
  line L4651 (-151.5449, 68.0838) -> (-152.3441, 68.0838)
  line L4652 (-61.858, 29.9838) -> (-61.858, 28.9833)
  line L4653 (-30.902, 0.7845) -> (-30.101, 0.7845)
  line L4654 (-61.858, 28.9833) -> (-61.858, 29.9838)
  line L4655 (-44.901, 4.8841) -> (-30.902, 4.8841)
  line L4656 (-152.3441, 71.1844) -> (-151.5449, 71.1844)
  line L4657 (-29.033, 10.9337) -> (-29.033, 14.0343)
  line L4658 (-152.3441, 81.084) -> (-166.345, 81.084)
  line L4659 (-126.1517, 0.7845) -> (-125.3512, 0.7845)
  line L4660 (-81.4205, 52.1344) -> (-81.4205, 49.0338)
  line L4661 (-18.195, 80.0836) -> (-18.994, 80.0836)
  line L4662 (-56.808, 28.9833) -> (-56.808, 29.9838)
  line L4663 (-85.6704, 52.1344) -> (-84.87, 52.1344)
  line L4664 (-30.101, 3.8837) -> (-30.101, 0.7845)
  line L4665 (-18.994, 81.084) -> (-18.994, 80.0836)
  line L4666 (-117.1378, -8.1163) -> (-117.1378, -5.0157)
  line L4667 (-57.608, 29.9838) -> (-57.608, 33.0844)
  line L4668 (-14.744, 76.9844) -> (-14.744, 80.0836)
  line L4669 (-14.744, 71.1844) -> (-13.945, 71.1844)
  line L4670 (-75.8576, 28.9833) -> (-61.858, 28.9833)
  line L4671 (-81.4205, 61.0336) -> (-81.4205, 57.9344)
  line L4672 (-116.3388, 4.8841) -> (-116.3388, 3.8837)
  line L4673 (-67.133, 14.0343) -> (-66.333, 14.0343)
  line L4674 (-84.5267, 0.1836) -> (-84.5267, 3.4138)
  line L4675 (-56.808, 29.9838) -> (-57.608, 29.9838)
  line L4676 (-116.3388, 0.7845) -> (-117.1378, 0.7845)
  line L4677 (-85.6704, 57.9344) -> (-84.87, 57.9344)
  line L4678 (-116.3388, -9.1167) -> (-116.3388, -8.1163)
  line L4679 (-13.945, 80.0836) -> (-13.945, 81.084)
  line L4680 (-86.2521, 4.3343) -> (-86.2521, 3.4138)
  line L4681 (-152.3441, 76.9844) -> (-152.3441, 71.1844)
  line L4682 (-152.3441, 71.1844) -> (-152.3441, 76.9844)
  line L4683 (-86.183, 10.9337) -> (-86.183, 14.0343)
  line L4684 (-67.133, 19.8345) -> (-66.333, 19.8345)
  line L4685 (-116.3388, -8.1163) -> (-116.3388, -9.1167)
  line L4686 (-84.5267, -8.8866) -> (-84.5267, -4.4162)
  line L4687 (-67.133, 14.0343) -> (-67.133, 10.9337)
  line L4688 (-30.902, 4.8841) -> (-44.901, 4.8841)
  line L4689 (-152.3441, 67.0833) -> (-152.3441, 68.0838)
  line L4690 (-85.3826, 10.9337) -> (-85.3826, 9.9333)
  line L4691 (-86.2521, -8.8866) -> (-84.5267, -8.8866)
  line L4692 (-66.333, 22.9336) -> (-67.133, 22.9336)
  line L4693 (-80.6201, 52.1344) -> (-81.4205, 52.1344)
  line L4694 (-84.87, 61.0336) -> (-84.87, 57.9344)
  line L4695 (-30.902, -5.0157) -> (-30.902, -4.4162)
  line L4696 (-85.3826, 9.9333) -> (-85.3826, 10.9337)
  line L4697 (-75.8576, 33.0844) -> (-75.8576, 38.8844)
  line L4698 (-125.3512, 0.7845) -> (-125.3512, 3.8837)
  line L4699 (-86.183, 14.0343) -> (-85.3826, 14.0343)
  line L4700 (-84.5267, -8.8866) -> (-86.2521, -8.8866)
  line L4701 (-84.5267, 3.4138) -> (-84.5267, 0.1836)
  line L4702 (-117.1378, 0.7845) -> (-117.1378, 3.8837)
  line L4703 (-81.4205, 57.9344) -> (-80.6201, 57.9344)
  line L4704 (-84.87, 57.9344) -> (-85.6704, 57.9344)
  line L4705 (-30.101, 3.8837) -> (-30.902, 3.8837)
  line L4706 (-61.858, 29.9838) -> (-61.057, 29.9838)
  line L4707 (-71.3829, 19.8345) -> (-70.582, 19.8345)
  line L4708 (-66.333, 23.934) -> (-66.333, 22.9336)
  line L4709 (-61.057, 29.9838) -> (-61.057, 33.0844)
  line L4710 (-116.3388, 0.7845) -> (-116.3388, -5.0157)
  line L4711 (-86.2521, 3.4138) -> (-84.5267, 3.4138)
  line L4712 (-116.3388, 3.8837) -> (-117.1378, 3.8837)
  line L4713 (-81.4205, 57.9344) -> (-81.4205, 61.0336)
  line L4714 (-86.2521, -9.8664) -> (-86.2521, -8.8866)
  line L4715 (-67.133, 22.9336) -> (-66.333, 22.9336)
  line L4716 (-84.5267, -4.4162) -> (-84.5267, -8.8866)
  line L4717 (-86.183, 22.9336) -> (-86.183, 19.8345)
  line L4718 (-66.333, 10.9337) -> (-66.333, 9.9333)
  line L4719 (-80.6201, 61.0336) -> (-81.4205, 61.0336)
  line L4720 (-86.183, 19.8345) -> (-86.183, 22.9336)
  line L4721 (-86.183, 19.8345) -> (-85.3826, 19.8345)
  line L4722 (-70.582, 14.0343) -> (-70.582, 10.9337)
  line L4723 (-117.1378, -5.0157) -> (-116.3388, -5.0157)
  line L4724 (-56.808, 29.9838) -> (-56.808, 28.9833)
  line L4725 (-71.3829, 22.9336) -> (-70.582, 22.9336)
  line L4726 (-57.608, 33.0844) -> (-57.608, 29.9838)
  line L4727 (-86.2521, -8.8866) -> (-86.2521, -9.8664)
  line L4728 (-116.3388, -8.1163) -> (-117.1378, -8.1163)
  line L4729 (-70.582, 22.9336) -> (-71.3829, 22.9336)
  line L4730 (-86.183, 10.9337) -> (-85.3826, 10.9337)
  line L4731 (-71.3829, 9.9333) -> (-85.3826, 9.9333)
  arc A71 (-81.201, -13.9426) -> (-83.201, -15.9426) centre (-81.201, -15.9426) ccw
  line L4732 (-66.333, 9.9333) -> (-66.333, 10.9337)
  line L4733 (-30.101, -8.1163) -> (-30.902, -8.1163)
  line L4734 (-70.582, 14.0343) -> (-71.3829, 14.0343)
  line L4735 (-30.902, 3.8837) -> (-30.101, 3.8837)
  line L4736 (-85.3826, 22.9336) -> (-86.183, 22.9336)
  line L4737 (-66.333, 14.0343) -> (-67.133, 14.0343)
  line L4738 (-81.4205, 49.0338) -> (-81.4205, 52.1344)
  line L4739 (-80.6201, 48.0333) -> (-80.6201, 49.0338)
  line L4740 (-80.6201, 49.0338) -> (-81.4205, 49.0338)
  line L4741 (-66.333, 22.9336) -> (-66.333, 23.934)
  line L4742 (-86.183, 22.9336) -> (-85.3826, 22.9336)
  line L4743 (-80.1075, 29.9838) -> (-80.9079, 29.9838)
  line L4744 (-81.4205, 49.0338) -> (-80.6201, 49.0338)
  line L4745 (-61.057, 29.9838) -> (-61.858, 29.9838)
  line L4746 (-44.901, -9.1167) -> (-30.902, -9.1167)
  line L4747 (-30.101, -5.0157) -> (-30.902, -5.0157)
  line L4748 (-75.8576, 29.9838) -> (-75.8576, 28.9833)
  line L4749 (-30.902, -4.4162) -> (-30.902, -5.0157)
  line L4750 (-85.3826, 23.934) -> (-85.3826, 22.9336)
  line L4751 (-71.3829, 23.934) -> (-71.3829, 22.9336)
  line L4752 (-30.902, 4.8841) -> (-30.902, 3.8837)
  line L4753 (-80.9079, 41.9836) -> (-80.9079, 42.984)
  line L4754 (-30.902, 0.7845) -> (-30.902, 0.1836)
  line L4755 (-76.658, 29.9838) -> (-75.8576, 29.9838)
  line L4756 (-67.133, 10.9337) -> (-66.333, 10.9337)
  line L4757 (-71.3829, 23.934) -> (-85.3826, 23.934)
  line L4758 (-71.3829, 22.9336) -> (-71.3829, 23.934)
  line L4759 (-75.8576, 28.9833) -> (-75.8576, 29.9838)
  line L4760 (-47.283, 9.9333) -> (-33.283, 9.9333)
  line L4761 (-76.658, 38.8844) -> (-76.658, 41.9836)
  line L4762 (-75.8576, 29.9838) -> (-76.658, 29.9838)
  line L4763 (-70.582, 19.8345) -> (-71.3829, 19.8345)
  line L4764 (-70.582, 19.8345) -> (-70.582, 22.9336)
  line L4765 (-85.3826, 23.934) -> (-71.3829, 23.934)
  line L4766 (-85.3826, 14.0343) -> (-86.183, 14.0343)
  line L4767 (-75.8576, 38.8844) -> (-76.658, 38.8844)
  line L4768 (-70.582, 10.9337) -> (-70.582, 14.0343)
  line L4769 (-71.3829, 14.0343) -> (-70.582, 14.0343)
  line L4770 (-85.3826, 9.9333) -> (-71.3829, 9.9333)
  line L4771 (-80.9079, 28.9833) -> (-80.9079, 29.9838)
  line L4772 (-71.3829, 10.9337) -> (-70.582, 10.9337)
  line L4773 (-85.3826, 19.8345) -> (-86.183, 19.8345)
  line L4774 (-76.658, 33.0844) -> (-75.8576, 33.0844)
  line L4775 (-75.8576, 33.0844) -> (-76.658, 33.0844)
  line L4776 (-85.3826, 10.9337) -> (-86.183, 10.9337)
  line L4777 (-85.3826, 22.9336) -> (-85.3826, 23.934)
  line L4778 (-48.083, 10.9337) -> (-47.283, 10.9337)
  line L4779 (-71.3829, 9.9333) -> (-71.3829, 10.9337)
  line L4780 (-47.283, 10.9337) -> (-47.283, 9.9333)
  line L4781 (-75.8576, 38.8844) -> (-75.8576, 33.0844)
  line L4782 (-30.902, -9.1167) -> (-30.902, -8.1163)
  line L4783 (-30.902, -8.1163) -> (-30.902, -9.1167)
  line L4784 (-80.1075, 41.9836) -> (-80.1075, 38.8844)
  line L4785 (-66.333, 10.9337) -> (-67.133, 10.9337)
  line L4786 (-70.582, 22.9336) -> (-70.582, 19.8345)
  line L4787 (-76.658, 33.0844) -> (-76.658, 29.9838)
  line L4788 (-47.283, 10.9337) -> (-48.083, 10.9337)
  line L4789 (-80.9079, 29.9838) -> (-80.1075, 29.9838)
  line L4790 (-80.9079, 38.8844) -> (-80.1075, 38.8844)
  line L4791 (-30.101, 0.7845) -> (-30.902, 0.7845)
  line L4792 (-75.8576, 41.9836) -> (-75.8576, 42.984)
  line L4793 (-80.9079, 33.0844) -> (-80.9079, 38.8844)
  line L4794 (-86.183, 14.0343) -> (-86.183, 10.9337)
  line L4795 (-71.3829, 10.9337) -> (-71.3829, 9.9333)
  line L4796 (-80.1075, 38.8844) -> (-80.1075, 41.9836)
  line L4797 (-30.902, -9.1167) -> (-44.901, -9.1167)
  line L4798 (-80.1075, 33.0844) -> (-80.9079, 33.0844)
  line L4799 (-51.532, 10.9337) -> (-51.532, 14.0343)
  line L4800 (-45.702, -5.0157) -> (-44.901, -5.0157)
  line L4801 (-80.9079, 33.0844) -> (-80.1075, 33.0844)
  line L4802 (-80.1075, 29.9838) -> (-80.1075, 33.0844)
  line L4803 (-76.658, 41.9836) -> (-75.8576, 41.9836)
  line L4804 (-75.8576, 42.984) -> (-75.8576, 41.9836)
  line L4805 (-51.532, 14.0343) -> (-51.532, 10.9337)
  line L4806 (-33.283, 9.9333) -> (-33.283, 10.9337)
  line L4807 (-76.658, 38.8844) -> (-75.8576, 38.8844)
  line L4808 (-45.702, 3.8837) -> (-44.901, 3.8837)
  line L4809 (-80.9079, 29.9838) -> (-80.9079, 28.9833)
  line L4810 (-76.658, 41.9836) -> (-76.658, 38.8844)
  line L4811 (-80.9079, 42.984) -> (-80.9079, 41.9836)
  line L4812 (-44.901, -5.0157) -> (-44.901, -4.4162)
  line L4813 (-76.658, 29.9838) -> (-76.658, 33.0844)
  line L4814 (-80.1075, 41.9836) -> (-80.9079, 41.9836)
  line L4815 (-80.9079, 38.8844) -> (-80.9079, 33.0844)
  line L4816 (-33.283, 14.0343) -> (-32.482, 14.0343)
  line L4817 (-33.283, 10.9337) -> (-33.283, 9.9333)
  line L4818 (-33.283, 10.9337) -> (-32.482, 10.9337)
  line L4819 (-51.532, 10.9337) -> (-52.333, 10.9337)
  line L4820 (-80.1075, 33.0844) -> (-80.1075, 29.9838)
  line L4821 (-52.333, 10.9337) -> (-52.333, 9.9333)
  line L4822 (-80.9079, 41.9836) -> (-80.1075, 41.9836)
  line L4823 (-80.1075, 38.8844) -> (-80.9079, 38.8844)
  line L4824 (-51.532, 14.0343) -> (-52.333, 14.0343)
  line L4825 (-44.901, -5.0157) -> (-45.702, -5.0157)
  line L4826 (-52.333, 14.0343) -> (-51.532, 14.0343)
  line L4827 (-44.901, -9.1167) -> (-44.901, -8.1163)
  line L4828 (-75.8576, 41.9836) -> (-76.658, 41.9836)
  line L4829 (-44.901, -8.1163) -> (-45.702, -8.1163)
  line L4830 (-52.333, 10.9337) -> (-51.532, 10.9337)
  line L4831 (-47.283, 9.9333) -> (-47.283, 10.9337)
  line L4832 (-33.283, 9.9333) -> (-47.283, 9.9333)
  line L4833 (-44.901, 0.7845) -> (-45.702, 0.7845)
  line L4834 (-45.702, 3.8837) -> (-45.702, 0.7845)
  line L4835 (-32.482, 10.9337) -> (-32.482, 14.0343)
  point P0 (-171.164, -14.1328)
  dimension "d135" = 3.4
  dimension "d136" = 3.4
  dimension "d137" = 50
  dimension "d138" = 3.4
  dimension "d139" = 50
  dimension "d140" = 3.4
  dimension "d141" = 3.4
  dimension "d142" = 7
  dimension "d143" = 3.4
  dimension "d144" = 3.4
  dimension "d145" = 2
  dimension "d146" = 3.4
  dimension "d147" = 3.4
  dimension "d148" = 60
  dimension "d149" = 3.4
  dimension "d150" = 3.4
  dimension "d151" = 60
  dimension "d152" = 3.4
  dimension "d153" = 3.4
  dimension "d154" = 3.4
  dimension "d155" = 3.4
  dimension "d156" = 3.4
  dimension "d157" = 3.4
  dimension "d158" = 3.4
  dimension "d159" = 3.4
  dimension "d160" = 3.4
  dimension "d161" = 3.4
  dimension "d162" = 3.4
  dimension "d163" = 3.4
  dimension "d164" = 3.4
  dimension "d165" = 3.4
  dimension "d166" = 11.7
  dimension "d167" = 11.7
  dimension "d168" = 11.7
  dimension "d169" = 11.7
  dimension "d170" = 11.7
  dimension "d171" = 11.7
  dimension "d172" = 11.7
  dimension "d173" = 11.7
  dimension "d174" = 11.7
  dimension "d175" = 11.7
  dimension "d176" = 11.7
  dimension "d177" = 11.7
  dimension "d178" = 11.7
  dimension "d179" = 11.7
  dimension "d180" = 11.7
  dimension "d181" = 11.7
  dimension "d182" = 11.7
  dimension "d183" = 11.7
  dimension "d184" = 11.7
  dimension "d185" = 11.7
  dimension "d186" = 11.7
  dimension "d187" = 11.7
  dimension "d188" = 2
  dimension "d189" = 12
  dimension "d190" = 11.7
  dimension "d191" = 0.5
  dimension "d192" = 0.5
  dimension "d193" = 0.5
  dimension "d194" = 0.5
  dimension "d195" = 9.541
  dimension "d196" = 4.801
  constraint horizontal L1825
  constraint horizontal L794
  constraint perpendicular L4112 L4158
  constraint perpendicular L3336 L4363
  constraint perpendicular L1441 L1475
  constraint perpendicular L1455 L1488
  constraint collinear L1652 L4388
  constraint collinear L1652 L3231
  constraint collinear L1385 L3231
  constraint collinear L1385 L2614
  constraint collinear L794 L2614
  constraint collinear L1048 L1102
  constraint collinear L207 L1048
  constraint collinear L207 L3271
  constraint collinear L1099 L3271
  constraint collinear L1099 L1825
  constraint collinear L1455 L1475
  constraint collinear L1473 L1475
  constraint collinear L6 L1473
  constraint collinear L6 L904
  constraint collinear L904 L1147
  constraint collinear L1106 L1147
  constraint collinear L739 L1493
  constraint collinear L926 L1493
  constraint collinear L796 L926
  constraint perpendicular L21 L1414
  constraint collinear L796 L3336
  constraint collinear L3336 L4112
  constraint tangent A32 L1488
  constraint tangent A32 L1455
  constraint tangent A38 L1488
  constraint tangent A38 L1825
  constraint equal A32 A38
  constraint tangent A33 L1825
  constraint tangent A33 L1441
  constraint equal A32 A33
  constraint tangent L1441 A40
  constraint tangent A40 L1475
  constraint equal A32 A40
  constraint tangent A35 L1475
  constraint tangent A35 L1477
  constraint equal A32 A35
  constraint tangent A34 L1477
  constraint tangent L1099 A34
  constraint equal A32 A34
  constraint tangent L1099 A70
  constraint tangent L4631 A70
  constraint equal A32 A70
  constraint tangent L4631 A71
  constraint tangent L1473 A71
  constraint equal A32 A71
  constraint tangent L1473 A48
  constraint tangent A48 L3199
  constraint equal A32 A48
  constraint tangent L3199 A55
  constraint tangent A55 L3271
  constraint equal A32 A55
  constraint tangent A44 L3271
  constraint tangent L2428 A44
  constraint equal A32 A44
  constraint tangent L2428 A46
  constraint tangent L6 A46
  constraint equal A32 A46
  constraint tangent L6 A13
  constraint tangent A13 L871
  constraint equal A13 A32
  constraint tangent A12 L871
  constraint tangent L207 A12
  constraint equal A12 A32
  constraint tangent L207 A1
  constraint tangent L205 A1
  constraint equal A1 A32
  constraint tangent L205 A3
  constraint tangent A3 L904
  constraint equal A3 A32
  constraint tangent L904 A31
  constraint tangent L1105 A31
  constraint equal A31 A32
  constraint tangent A16 L1105
  constraint tangent L1048 A16
  constraint equal A16 A32
  constraint tangent L1048 A27
  constraint tangent L1134 A27
  constraint equal A27 A32
  constraint tangent A22 L1134
  constraint tangent A22 L1147
  constraint equal A22 A32
  constraint tangent A23 L1147
  constraint tangent L1079 A23
  constraint equal A23 A32
  constraint tangent L1079 A28
  constraint tangent L1102 A28
  constraint equal A28 A32
  constraint tangent L1070 A30
  constraint tangent L1102 A30
  constraint equal A30 A32
  constraint tangent L1070 A19
  constraint tangent A19 L1106
  constraint equal A19 A32
  constraint tangent L761 A10
  constraint tangent L739 A10
  constraint equal A10 A32
  constraint tangent L761 A8
  constraint tangent A8 L794
  constraint equal A8 A32
  constraint tangent L729 A7
  constraint tangent A7 L794
  constraint equal A7 A32
  constraint tangent L729 A6
  constraint tangent A6 L1493
  constraint equal A6 A32
  constraint tangent A45 L2522
  constraint tangent L1493 A45
  constraint equal A32 A45
  constraint tangent A42 L2522
  constraint tangent A42 L2614
  constraint equal A32 A42
  constraint tangent A4 L577
  constraint tangent A4 L2614
  constraint equal A4 A32
  constraint tangent L577 A11
  constraint tangent A11 L926
  constraint equal A11 A32
  constraint tangent A14 L1372
  constraint tangent L926 A14
  constraint equal A14 A32
  constraint tangent A20 L1372
  constraint tangent A20 L1385
  constraint equal A20 A32
  constraint tangent A24 L1414
  constraint tangent A24 L1385
  constraint equal A24 A32
  constraint tangent A26 L1414
  constraint tangent L21 A26
  constraint equal A26 A32
  constraint tangent L3768 A62
  constraint tangent L21 A62
  constraint equal A32 A62
  constraint tangent A61 L3768
  constraint tangent L3231 A61
  constraint equal A32 A61
  constraint tangent A56 L3636
  constraint tangent L3231 A56
  constraint equal A32 A56
  constraint tangent A57 L3636
  constraint tangent L796 A57
  constraint equal A32 A57
  constraint tangent L3488 A58
  constraint tangent L796 A58
  constraint equal A32 A58
  constraint tangent L3488 A59
  constraint tangent L1652 A59
  constraint equal A32 A59
  constraint tangent A51 L3076
  constraint tangent L1652 A51
  constraint equal A32 A51
  constraint tangent A52 L3076
  constraint tangent A52 L3336
  constraint equal A32 A52
  constraint tangent L4363 A67
  constraint tangent L3336 A67
  constraint equal A32 A67
  constraint tangent A64 L4363
  constraint tangent A64 L4388
  constraint equal A32 A64